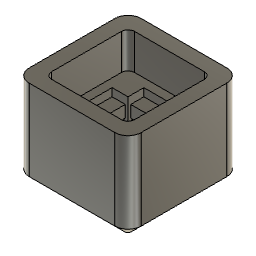
gds_pockettype_key (Autodesk Fusion 360 design; units mm, degrees)
Autodesk Fusion 360 part; units mm, degrees
sketch "Sketch1" plane through (0, 0, 0) normal (0, 0, 1) x (1, 0, 0)
  line L0 (3.25, -4.25) -> (-3.25, -4.25)
  line L1 (-4.25, -3.25) -> (-4.25, 3.25)
  line L2 (-3.25, 4.25) -> (3.25, 4.25)
  line L3 (4.25, 3.25) -> (4.25, -3.25)
  line L4 (4.25, -4.25) -> (-4.25, 4.25) construction
  line L5 (-4.25, -4.25) -> (4.25, 4.25) construction
  arc A0 (-3.25, 4.25) -> (-4.25, 3.25) centre (-3.25, 3.25) ccw
  arc A1 (4.25, 3.25) -> (3.25, 4.25) centre (3.25, 3.25) ccw
  arc A2 (3.25, -4.25) -> (4.25, -3.25) centre (3.25, -3.25) ccw
  arc A3 (-4.25, -3.25) -> (-3.25, -4.25) centre (-3.25, -3.25) ccw
  line L6 (0, 4.25) -> (0, -4.25)
  line L7 (4.25, 0) -> (-4.25, 0)
  line L8 (-2.65, 3.15) -> (2.65, 3.15)
  line L9 (3.15, 2.65) -> (3.15, -2.65)
  line L10 (2.65, -3.15) -> (-2.65, -3.15)
  line L11 (-3.15, -2.65) -> (-3.15, 2.65)
  line L12 (-3.15, 3.15) -> (3.15, -3.15) construction
  line L13 (3.15, 3.15) -> (-3.15, -3.15) construction
  arc A4 (-2.65, 3.15) -> (-3.15, 2.65) centre (-2.65, 2.65) ccw
  arc A5 (3.15, 2.65) -> (2.65, 3.15) centre (2.65, 2.65) ccw
  arc A6 (-3.15, -2.65) -> (-2.65, -3.15) centre (-2.65, -2.65) ccw
  arc A7 (2.65, -3.15) -> (3.15, -2.65) centre (2.65, -2.65) ccw
  circle A8 centre (0, 0) radius 1
  line L14 (1.3, 1.3) -> (-1.3, 1.3)
  line L15 (-1.3, 1.3) -> (-1.3, -1.3)
  line L16 (-1.3, -1.3) -> (1.3, -1.3)
  line L17 (1.3, -1.3) -> (1.3, 1.3)
  line L18 (1.3, 1.3) -> (-1.3, -1.3) construction
  line L19 (-1.3, 1.3) -> (1.3, -1.3) construction
  point P0 (0, 2.3)
  dimension "d1" = 8.5
  dimension "d4" = 1
  dimension "d5" = 1
  dimension "d6" = 1
  dimension "d7" = 1
  dimension "d15" = 6.3
  dimension "d16" = 0.5
  dimension "d17" = 0.5
  dimension "d18" = 0.5
  dimension "d19" = 0.5
  dimension "d40" = 2
  dimension "d57" = 2.6
  constraint horizontal L0
  constraint perpendicular L0 L1
  constraint parallel L0 L2
  constraint parallel L1 L3
  constraint coincident L4 A8.centre
  constraint coincident L5 A8.centre
  constraint coincident A8.centre origin
  constraint coincident L4.end L1
  constraint coincident L4.end L2
  constraint tangent L1 A0
  constraint tangent L2 A0
  constraint coincident L5.end L3
  constraint coincident L5.end L2
  constraint tangent L3 A1
  constraint tangent L2 A1
  constraint coincident L4.start L3
  constraint coincident L4.start L0
  constraint tangent L3 A2
  constraint tangent L0 A2
  constraint coincident L5.start L0
  constraint coincident L5.start L1
  constraint tangent L0 A3
  constraint tangent L1 A3
  constraint equal L1 L2
  constraint midpoint L2 L6.start
  constraint midpoint L0 L6.end
  constraint midpoint L3 L7.start
  constraint midpoint L1 L7.end
  constraint coincident P0 L6
  constraint horizontal L8
  constraint perpendicular L8 L9
  constraint parallel L8 L10
  constraint parallel L9 L11
  constraint coincident L4 L12.start
  constraint coincident L12 A8.centre
  constraint coincident L13 A8.centre
  constraint coincident L12.start L8
  constraint coincident L12.start L11
  constraint tangent L8 A4
  constraint tangent L11 A4
  constraint coincident L13.start L8
  constraint coincident L13.start L9
  constraint tangent L8 A5
  constraint tangent L9 A5
  constraint coincident L13.end L11
  constraint coincident L13.end L10
  constraint tangent L11 A6
  constraint tangent L10 A6
  constraint coincident L12.end L10
  constraint coincident L12.end L9
  constraint tangent L10 A7
  constraint tangent L9 A7
  constraint horizontal L14
  constraint perpendicular L14 L15
  constraint parallel L14 L16
  constraint parallel L15 L17
  constraint coincident L5 L14.start
  constraint coincident L18 A8.centre
  constraint coincident L19 A8.centre
  constraint coincident L15.start L14
  constraint coincident L14.end L15
  constraint coincident L17.end L14
  constraint coincident L14.start L17
  constraint coincident L16.end L17
  constraint coincident L17.start L16
  constraint coincident L16.start L15
  constraint coincident L15.end L16
  constraint coincident L14.end L15.start
  constraint coincident L14.start L17.end
  constraint coincident L16.end L17.start
  constraint coincident L15.end L16.start
  measures "d1" distance of L0 L2
  measures "d4" radius of A0
  measures "d5" radius of A1
  measures "d6" radius of A2
  measures "d7" radius of A3
  measures "d15" distance of L9 L11
  measures "d16" radius of A4
  measures "d17" radius of A5
  measures "d18" radius of A6
  measures "d19" radius of A7
  measures "d40" diameter of A8
  measures "d57" distance of L15 L17
extrude "Extrude1" add sketch "Sketch1" along normal blind 6.9
extrude "Extrude2" cut sketch "Sketch1" along normal up to surface (5.9 mm away) from surface at 1 contours L6 L7 L10 L11 A6 L15 L16 | L6 L7 L9 L10 A7 L16 L17 | L6 L7 A8 L15 L16 | L6 L7 A8 L16 L17 | L6 L7 L8 L9 A5 L14 L17 | L6 L7 A8 | L6 L7 A8 | L6 L7 A8 L14 L17 | L6 L7 L8 L11 A4 L14 L15 | L6 L7 A8 | L6 L7 A8 | L6 L7 A8 L14 L15
chamfer "Chamfer1" distance 0.75 angle 45 8 edges at (-4.25, 0, 0) (-3.9571, 3.9571, 0) (0, 4.25, 0) (3.9571, 3.9571, 0) (4.25, 0, 0) (3.9571, -3.9571, 0) (0, -4.25, 0) (-3.9571, -3.9571, 0)
extrude "Extrude4" add sketch "Sketch1" along normal blind 2.9 from surface at 1 contours L6 L7 L10 L11 A6 L15 L16 | L6 L7 L9 L10 A7 L16 L17 | L6 L7 L8 L9 A5 L14 L17 | L6 L7 L8 L11 A4 L14 L15
sketch "Sketch3" plane through (0, 0, 3.9) normal (0, 0, 1) x (-1, 0, 0)
  line L0 (-1.3, -1.3) -> (-1.3, 1.3)
  line L1 (-1.3, 1.3) -> (1.3, 1.3)
  line L2 (1.3, 1.3) -> (1.3, -1.3)
  line L3 (1.3, -1.3) -> (-1.3, -1.3)
  arc A0 (3.15, 2.65) -> (2.65, 3.15) centre (2.65, 2.65) ccw
  line L4 (2.65, 3.15) -> (-2.65, 3.15)
  arc A1 (-2.65, 3.15) -> (-3.15, 2.65) centre (-2.65, 2.65) ccw
  line L5 (-3.15, 2.65) -> (-3.15, -2.65)
  arc A2 (-3.15, -2.65) -> (-2.65, -3.15) centre (-2.65, -2.65) ccw
  line L6 (-2.65, -3.15) -> (2.65, -3.15)
  arc A3 (2.65, -3.15) -> (3.15, -2.65) centre (2.65, -2.65) ccw
  line L7 (3.15, -2.65) -> (3.15, 2.65)
  line L8 (1.3, -1.3) -> (1.3, -2.5052)
  line L9 (1.3, -2.5052) -> (-1.3, -2.5052)
  line L10 (-1.3, -2.5052) -> (-1.3, -1.3)
  line L11 (-1, -1.3) -> (-1, -2.2052)
  line L12 (-1, -2.2052) -> (1, -2.2052)
  line L13 (1, -2.2052) -> (1, -1.3)
  line L14 (1.3, -1) -> (2.2052, -1)
  line L15 (2.5052, -1.3) -> (1.3, -1.3)
  line L16 (2.2052, 1) -> (1.3, 1)
  line L17 (1.3, 1.3) -> (1.3, -1.3)
  line L18 (1.3, 1.3) -> (2.5052, 1.3)
  line L19 (2.2052, -1) -> (2.2052, 1)
  line L20 (2.5052, 1.3) -> (2.5052, -1.3)
  line L21 (1, 1.3) -> (1, 2.2052)
  line L22 (1.3, 2.5052) -> (1.3, 1.3)
  line L23 (-1, 2.2052) -> (-1, 1.3)
  line L24 (-1.3, 1.3) -> (1.3, 1.3)
  line L25 (-1.3, 1.3) -> (-1.3, 2.5052)
  line L26 (1, 2.2052) -> (-1, 2.2052)
  line L27 (-1.3, 2.5052) -> (1.3, 2.5052)
  line L28 (-1.3, 1) -> (-2.2052, 1)
  line L29 (-2.5052, 1.3) -> (-1.3, 1.3)
  line L30 (-2.2052, -1) -> (-1.3, -1)
  line L31 (-1.3, -1.3) -> (-1.3, 1.3)
  line L32 (-1.3, -1.3) -> (-2.5052, -1.3)
  line L33 (-2.2052, 1) -> (-2.2052, -1)
  line L34 (-2.5052, -1.3) -> (-2.5052, 1.3)
  line L35 (1, -1.3) -> (-1, -1.3)
  line L36 (-1, -1.3) -> (-1, -1.2)
  line L37 (-1, -1.2) -> (1, -1.2)
  line L38 (1, -1.2) -> (1, -1.3)
  line L39 (1.2, 1) -> (1.3, 1)
  line L40 (1.2, -1) -> (1.2, 1)
  line L41 (1.3, -1) -> (1.2, -1)
  line L42 (-1, 1.2) -> (-1, 1.3)
  line L43 (1, 1.2) -> (-1, 1.2)
  line L44 (1, 1.3) -> (1, 1.2)
  line L45 (-1.2, -1) -> (-1.3, -1)
  line L46 (-1.2, 1) -> (-1.2, -1)
  line L47 (-1.3, 1) -> (-1.2, 1)
  dimension "d50" = 0.3
  dimension "d51" = 0.3
  dimension "d52" = 0.3
  dimension "d54" = 360
  dimension "d58" = 0.1
  constraint coincident L2.end L3.start
  constraint perpendicular L3 L8
  constraint perpendicular L8 L9
  constraint coincident L0.start L3.end
  constraint perpendicular L9 L10
  constraint vertical L11
  constraint horizontal L12
  constraint vertical L13
  constraint coincident L3 L13.end
  constraint coincident L3 L11.start
  constraint horizontal L35
  constraint vertical L36
  constraint horizontal L37
  constraint vertical L38
  constraint coincident L11.start L35.end
  measures "d50" distance of L8 L13
  measures "d51" distance of L10 L11
  measures "d52" distance of L9 L12
  measures "d58" distance of L35 L37
extrude "Extrude5" cut sketch "Sketch3" against normal up to surface (2.9 mm away) contours L0 L28 L29 L30 L31 L32 L33 L34 | L3 L8 L9 L10 L11 L12 L13 | L1 L21 L22 L23 L24 L25 L26 L27 | L2 L14 L15 L16 L17 L18 L19 L20
extrude "Extrude6" add sketch "Sketch3" against normal blind 0.9 contours L0 L31 L45 L46 L47 | L3 L35 L36 L37 L38 | L1 L24 L42 L43 L44 | L2 L17 L39 L40 L41
extrude "Extrude8" add sketch "Sketch3" along normal blind 0.3
extrude "Extrude7" [suppressed]
fillet "Fillet2" [suppressed]
equation "d1 = KeyFaceSize"
equation "KeyFaceSize = 8.5 mm"
equation "CornerRadius = 1 mm"
equation "d4 = CornerRadius"
equation "d5 = CornerRadius"
equation "d6 = CornerRadius"
equation "d7 = CornerRadius"
equation "StemSize = 2.6 mm"
equation "InnerSize = 6.3 mm"
equation "d15 = InnerSize"
equation "KeyFaceThickness = 1 mm"
equation "d46 = KeyFaceThickness"
equation "d57 = StemSize"
